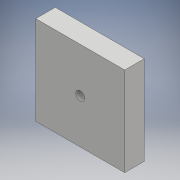
# Autodesk Inventor part: peltier_41x41x9
Saved by Autodesk Inventor 2018 (Build 220112000, 112)
## iProperties
Created: 2017-11-18
Part Number: peltier_41x41x9
Material: Generic
Document SubType Name: Modeling
Designer: MISAKA
Density: 1 g/cm^3
Appearance: Default
Author: MISAKA
Autodesk Inventor part; units mm, degrees
ref_plane "YZ Plane" through (0, 0, 0) normal (1, 0, 0) x (0, 1, 0)
ref_plane "XZ Plane" through (0, 0, 0) normal (0, 1, 0) x (-1, 0, 0)
ref_plane "XY Plane" through (0, 0, 0) normal (0, 0, 1) x (1, 0, 0)
sketch "Sketch1" plane through (0, 0, 0) normal (0, 1, 0) x (-1, 0, 0)
  line L0 (-20.5, 20.5) -> (20.5, 20.5)
  line L1 (20.5, 20.5) -> (20.5, -20.5)
  line L2 (20.5, -20.5) -> (-20.5, -20.5)
  line L3 (-20.5, -20.5) -> (-20.5, 20.5)
  line L4 (-20.5, 20.5) -> (20.5, -20.5) construction
  line L5 (20.5, 20.5) -> (-20.5, -20.5) construction
  circle A0 centre (0, 0) radius 2
  dimension "d0" = 41
  dimension "d1" = 4
  constraints: 12 end point, 2 midpoint, 2 parallel, 2 perpendicular, 1 centre point, 1 coincident, 1 horizontal
  measures "d0" distance of L0.end L1.end
  measures "d1" diameter of A0
extrude "Extrusion1" add sketch "Sketch1" along normal blind 9
body "Solid1"
